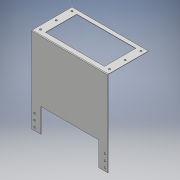
# Autodesk Inventor part: psu mount
Saved by Autodesk Inventor 2018 (Build 220112000, 112)
## iProperties
Created: 2018-06-20
Part Number: psu mount
Material: Generic
Document SubType Name: Sheet Metal
Designer: John Viljoen
Density: 1 g/cm^3
Sheet Metal Rule: Default_mm
Appearance: Default
Author: John Viljoen
Autodesk Inventor part; units mm, degrees
ref_plane "YZ Plane" through (0, 0, 0) normal (1, 0, 0) x (0, 1, 0)
ref_plane "XZ Plane" through (0, 0, 0) normal (0, 1, 0) x (-1, 0, 0)
ref_plane "XY Plane" through (0, 0, 0) normal (0, 0, 1) x (1, 0, 0)
sketch "Sketch1" plane through (0, 0, 0) normal (0, 0, 1) x (1, 0, 0)
  line L0 (0, 0) -> (125, 0)
  line L1 (125, 0) -> (125, 64)
  line L2 (125, 64) -> (0, 64)
  line L3 (0, 64) -> (0, 0)
  line L4 (0, 64) -> (14.15, 64) construction
  line L5 (14.15, 64) -> (14.15, 57.7) construction
  line L6 (14.15, 57.7) -> (110.85, 57.7)
  line L7 (110.85, 57.7) -> (110.85, 6.3)
  line L8 (110.85, 6.3) -> (14.15, 6.3)
  line L9 (14.15, 6.3) -> (14.15, 57.7)
  line L10 (0, 64) -> (0, 57.85) construction
  line L11 (0, 57.85) -> (6, 57.85) construction
  line L12 (6, 57.85) -> (6, 32.1) construction
  line L13 (6, 32.1) -> (6, 6.35) construction
  line L14 (6, 6.35) -> (119, 6.35) construction
  line L15 (119, 6.35) -> (119, 32.1) construction
  line L16 (119, 32.1) -> (119, 57.85) construction
  circle A0 centre (6, 57.85) radius 1.5
  circle A1 centre (6, 32.1) radius 1.5
  circle A2 centre (6, 6.35) radius 1.5
  circle A3 centre (119, 6.35) radius 1.5
  circle A4 centre (119, 57.85) radius 1.5
  circle A5 centre (119, 32.1) radius 1.5
  dimension "d0" = 125
  dimension "d1" = 64
  dimension "d2" = 14.15
  dimension "d3" = 6.3
  dimension "d4" = 96.7
  dimension "d5" = 51.4
  dimension "d6" = 6.15
  dimension "d7" = 6
  dimension "d8" = 25.75
  dimension "d9" = 25.75
  dimension "d10" = 113
  dimension "d11" = 3
  dimension "d12" = 3
  dimension "d13" = 3
  dimension "d14" = 3
  dimension "d16" = 3
  dimension "d18" = 3
  measures "d0" distance of L2.end L1.end
  measures "d1" distance of L1.end L0.end
  measures "d2" distance of L2.end L4.end
  measures "d3" distance of L4.end L5.end
  measures "d4" distance of L7.end L8.end
  measures "d5" distance of L6.end L7.end
  measures "d6" distance of L2.end L10.end
  measures "d7" distance of L10.end L11.end
  measures "d8" distance of L11.end L12.end
  measures "d9" distance of L12.end L13.end
  measures "d10" distance of L13.end L14.end
  measures "d11" diameter of A0
  measures "d12" diameter of A1
  measures "d13" diameter of A2
  measures "d14" diameter of A3
  measures "d16" diameter of A4
  measures "d18" diameter of A5
extrude "Plate2" add sketch "Sketch1" along normal blind 0.5
sketch "Sketch2" plane through (0, 0, 0.5) normal (0, 0, 1) x (1, 0, 0)
  line L0 (0, 0) -> (125, 0)
  line L1 (125, 0) -> (125, -1)
  line L2 (125, -1) -> (0, -1)
  line L3 (0, -1) -> (0, 0)
  dimension "d20" = 125
  dimension "d21" = 1
  measures "d20" distance of L1.end L2.end
  measures "d21" distance of L0.end L1.end
sheet face with bend "Face3" sketch "Sketch2" thickness 0.5 toward (0, 0, -1) bend radius 0.5
bend "Bend1"
sketch "Sketch4" plane through (0, -1, 0.5) normal (0, -1, 0) x (1, 0, 0)
  line L0 (0, -0.5) -> (125, -0.5) projected
  line L1 (125, 0) -> (125, -0.5) projected
  line L2 (0, 0) -> (125, 0) projected
  line L3 (0, 0) -> (0, -0.5) projected
extrude "Extrusion1" add sketch "Sketch4" along normal blind 1.15
sketch "Sketch5" plane through (0, -1.65, 0.5) normal (0, -1, 0) x (1, 0, 0)
  line L0 (125, 0) -> (0, 0)
  line L1 (0, 0) -> (0, -140)
  line L2 (0, -140) -> (125, -140)
  line L3 (125, -140) -> (125, 0)
  constraints: 6 end point, 1 horizontal, 1 perpendicular, 1 vertical
edge flange "Flange2" height 140 angle 90 thickness 0.5 bend radius 0.5 thickness toward (0, -1, 0) relief tear relief width 0.5 relief depth 0.25 edges at (62.5, -2.15, 0) wall of the first edge with corners at (125, -1.65, 0.5) (0, -1.65, 0.5) (0, -1.65, -139.5) (125, -1.65, -139.5)
bend "Bend3"
corner "Corner2"
sketch "Sketch6" plane through (0, -2.15, -139.5) normal (0, -1, 0) x (1, 0, 0)
  line L0 (0, 0) -> (0, 139) projected
  line L1 (125, 0) -> (0, 0) projected
  line L2 (125, 0) -> (120, 0) construction
  line L3 (120, 0) -> (120, 5) construction
  line L4 (120, 0) -> (110, 0) construction
  line L5 (110, 0) -> (110, 39.5) construction
  line L6 (110, 39.5) -> (15, 39.5) construction
  line L7 (15, 39.5) -> (110, 39.5)
  line L8 (110, 39.5) -> (110, 0)
  line L9 (110, 0) -> (15, 0)
  line L10 (15, 0) -> (15, 39.5)
  circle A0 centre (120, 5) radius 1.5
  line L11 (120, 5) -> (120, 15) construction
  line L12 (120, 15) -> (120, 25) construction
  circle A1 centre (120, 15) radius 1.5
  circle A2 centre (120, 25) radius 1.5
  line L13 (15, 0) -> (5, 0)
  circle A3 centre (5, 5) radius 1.5
  circle A4 centre (5, 15) radius 1.5
  circle A5 centre (5, 25) radius 1.5
  point P0 (0, 139.5)
  dimension "d49" = 5
  dimension "d50" = 5
  dimension "d51" = 10
  dimension "d52" = 39.5
  dimension "d53" = 95
  dimension "d54" = 3
  dimension "d55" = 10
  dimension "d56" = 10
  dimension "d57" = 3
  dimension "d58" = 3
  dimension "d59" = 10
  dimension "d60" = 3
  dimension "d61" = 3
  dimension "d62" = 3
  constraints: 24 end point, 6 centre point, 4 perpendicular, 4 point on line, 3 coincident, 2 parallel, 1 horizontal, 1 vertical
  measures "d49" distance of L1.start L2.end
  measures "d50" distance of L2.end L3.end
  measures "d51" distance of L2.end L4.end
  measures "d52" distance of L4.end L5.end
  measures "d53" distance of L5.end L6.end
  measures "d54" diameter of A0
  measures "d55" distance of L11.start L11.end
  measures "d56" distance of L11.end L12.end
  measures "d57" diameter of A1
  measures "d58" diameter of A2
  measures "d59" distance of L9.end L13.end
  measures "d60" diameter of A3
  measures "d61" diameter of A4
  measures "d62" diameter of A5
extrude "Extrusion2" cut sketch "Sketch6" against normal blind 1.15
equation "\"d19\" = Thickness"
equation "\"d22\" = BendRadius"
equation "\"d23\" = BendReliefWidth"
equation "\"d25\" = MinimumRemnant"
equation "\"d24\" = BendReliefDepth"
equation "\"d26\" = TransitionRadius"
equation "\"d39\" = BendReliefWidth"
equation "\"d40\" = BendReliefDepth"
equation "\"d41\" = MinimumRemnant"
equation "\"d42\" = TransitionRadius"
equation "\"d45\" = BendRadius"
equation "\"d46\" = CornerReliefSize"
equation "\"d47\" = GapSize"
equation "\"d48\" = JacobiRadiusSize"
equation "\"BendRadius\" = Thickness"
equation "\"BendReliefWidth\" = Thickness"
equation "\"BendReliefDepth\" = 0.5 * Thickness"
equation "\"CornerReliefSize\" = 4 * Thickness"
equation "\"MinimumRemnant\" = 2 * Thickness"
equation "\"TransitionRadius\" = BendRadius"
equation "\"JacobiRadiusSize\" = BendRadius"
equation "\"GapSize\" = Thickness"
equation "\"Thickness\" = 0.5"
body "Solid2"
